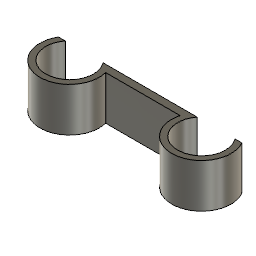
chassis (Autodesk Fusion 360 design; units mm, degrees)
Autodesk Fusion 360 part; units mm, degrees
sketch "スケッチ1" plane through (0, 0, 0) normal (0, 0, 1) x (1, 0, 0)
  arc A0 (-11.5217, 2) -> (-4.0754, 1) centre (-8, 0) ccw
  arc A1 (-10.5617, 2) -> (-5.4383, 2) centre (-8, 0) ccw
  line L0 (-11.5217, 2) -> (-10.5617, 2)
  line L1 (-6, 1) -> (-4.9077, 1)
  line L2 (-4.0754, 1) -> (6.0754, 1)
  arc A2 (6.0754, 1) -> (13.5217, 2) centre (10, 0) ccw
  arc A3 (7.4383, 2) -> (12.5617, 2) centre (10, 0) ccw
  line L3 (-5.4383, 2) -> (7.4383, 2)
  line L4 (12.5617, 2) -> (13.5217, 2)
  dimension "d7" = 6.5
  dimension "d8" = 6.5
  constraint horizontal L0
  constraint horizontal L1
  constraint concentric A0 A1
  constraint coincident A1.end L0
  constraint collinear L0 L3
  constraint coincident A1 L1.end
  constraint collinear L1 L2
  constraint concentric A2 A3
  constraint coincident A3.end L3
  constraint collinear L3 L4
  measures "d7" diameter of A1
  measures "d8" diameter of A3
extrude "押し出し3" add sketch "スケッチ1" along normal blind 6
extrude "押し出し2" [suppressed]
